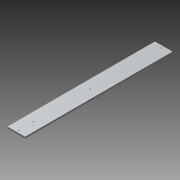
# Autodesk Inventor part: small side
Saved by Autodesk Inventor 2015 SP1 (Build 190203100, 203)
## iProperties
Created: 2015-01-31
Part Number: small side
Material: Generic
Document SubType Name: Modeling
Designer: Joseph
Density: 1 g/cm^3
Appearance: Default
Author: Joseph
Autodesk Inventor part; units mm, degrees
ref_plane "YZ Plane" through (0, 0, 0) normal (1, 0, 0) x (0, 1, 0)
ref_plane "XZ Plane" through (0, 0, 0) normal (0, 1, 0) x (-1, 0, 0)
ref_plane "XY Plane" through (0, 0, 0) normal (0, 0, 1) x (1, 0, 0)
sketch "Sketch1" plane through (0, 0, 0) normal (0, 0, 1) x (1, 0, 0)
  line L0 (0, 20) -> (25.8492, 20) projected
  line L1 (25.8492, 0) -> (25.8492, 20) projected
  line L2 (-45.8684, 0) -> (-45.8684, 20) projected
  line L3 (-20.0191, -580) -> (-45.8684, -580) projected
  line L4 (-45.8684, -580) -> (25.8492, -580)
  line L5 (25.8492, -580) -> (25.8492, 20)
  line L6 (25.8492, 20) -> (-45.8684, 20)
  line L7 (-45.8684, 20) -> (-45.8684, -580)
  point P0 (0, 0)
  constraints: 8 end point, 2 parallel, 1 horizontal, 1 perpendicular
extrude "Extrusion1" add sketch "Sketch1" along normal blind 6.35
sketch "Sketch2" plane through (0, 0, 6.35) normal (0, 0, 1) x (1, 0, 0)
  line L0 (25.8492, 20) -> (-45.8684, 20) projected
  line L1 (-45.8684, -580) -> (25.8492, -580) projected
  line L2 (-10.0096, 20) -> (-10.0096, -580) construction
  circle A0 centre (-10.0096, -580) radius 10 construction
  circle A1 centre (-10.0096, -580) radius 70 construction
  circle A2 centre (-10.0096, 20) radius 10 construction
  point P0 (0, 0)
  point P1 (-10.0096, -280)
  point P2 (-10.0096, -510)
  point P3 (-10.0096, -570)
  point P4 (-10.0096, 10)
  dimension "d2" = 20
  dimension "d3" = 140
  dimension "d4" = 20
  constraints: 3 coincident, 3 midpoint, 3 point on line, 3 vertical alignment, 2 end point, 6 other
hole "Hole1" at (-10.0096, -280, 6.35) at (-10.0096, -510, 6.35) at (-10.0096, -570, 6.35) at (-10.0096, 10, 6.35) direction (0, 0, -1) diameter 4.5 end through all clearance for "Socket Head Cap Screw" size "M4" standard "Ansi Metric M Profile"
body "Solid1"
